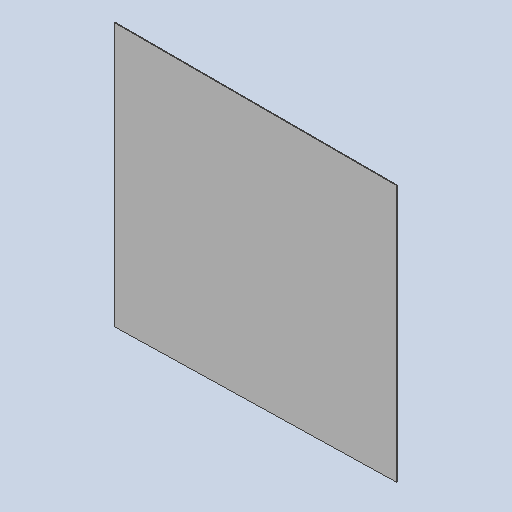
# Autodesk Inventor part: GBK 2311 shield 7
Saved by Autodesk Inventor 2026 (Build 300175000, 175)
## iProperties
Created: 2026-04-17
Part Number: GBK 2311 shield 7
Material: Steel
Document SubType Name: Sheet Metal
Designer: pokla
Stock Number: 2317
Mass: 69243.3 g
Surface Area: 44341.6 cm^2
Volume: 8820.8 cm^3
Density: 7.85 g/cm^3
Flat Pattern Width: 148 cm
Flat Pattern Length: 138.1 cm
Flat Pattern Area: 20438.8 cm^2
Sheet Metal Rule: По умолчанию_мм
Sheet Metal Width: 1480,000 мм
Sheet Metal Length: 1381,000 мм
Sheet Metal Area: 2043880,000 мм^2
Appearance: Default
Author: admin
Autodesk Inventor part; units mm, degrees
ref_plane "YZ Plane" through (0, 0, 0) normal (1, 0, 0) x (0, 1, 0)
ref_plane "XZ Plane" through (0, 0, 0) normal (0, 1, 0) x (-1, 0, 0)
ref_plane "XY Plane" through (0, 0, 0) normal (0, 0, 1) x (1, 0, 0)
sketch "Sketch1" plane through (0, 0, 0) normal (0, 0, 1) x (1, 0, 0)
  line L0 (740, -745) -> (-740, -745)
  line L1 (-740, -745) -> (-740, 745)
  line L2 (-740, 745) -> (740, 745)
  line L3 (740, 745) -> (740, -745)
  line L4 (740, -745) -> (-740, 745) construction
  line L5 (-740, -745) -> (740, 745) construction
  line L6 (-740, -636) -> (740, -602.4141)
  point P0 (0, 0)
  dimension "d0" = 1480
  dimension "d1" = 1490
  dimension "d4" = 1.3
  dimension "d9" = 1381
  dimension "d10" = 109
  measures "d0" distance of L1.end L2.end
  measures "d1" distance of L0.end L1.end
  measures "d4" angle of L0 L6
  measures "d9" distance of L1.end L6.start
  measures "d10" distance of L0.end L6.start
extrude "Plate1" add sketch "Sketch1" along normal blind 4 contours L6 L1 L2 L3
sketch "Эскиз3" plane through (0, 0, 0) normal (0, 0, -1) x (-1, 0, 0)
  line L0 (636.5062, -289.7957) -> (636.5062, -787.9319) construction
  line L1 (636.5062, -787.9319) -> (596.8789, -787.9319) construction
  line L2 (596.8789, -787.9319) -> (596.8789, -289.7957) construction
  line L3 (596.8789, -289.7957) -> (636.5062, -289.7957) construction
  line L4 (210.5058, -494) -> (210.5058, -591) projected
  line L5 (210.5058, -591) -> (206.5068, -591) projected
  line L6 (-289.6228, -494) -> (-289.6228, -591) projected
  line L7 (-289.6228, -591) -> (-293.6218, -591) projected
  line L8 (-739.3197, -490.5) -> (-710, -490.5) projected
  line L9 (-710, -490.5) -> (-710, -486.5) projected
  line L10 (-739.3197, 6.1667) -> (-710, 6.1667) projected
  line L11 (-710, 6.1667) -> (-710, 10.1667) projected
  line L12 (-739.3197, 502.8333) -> (-710, 502.8333) projected
  line L13 (-710, 502.8333) -> (-710, 506.8333) projected
  ellipse E0 centre (-289.6228, 744) end of major axis (-289.6228, 774) minor radius 0.6803 (-289.6228, 714) -> (-289.6228, 774) ccw projected
  line L14 (-289.6228, 714) -> (-293.6218, 714) projected
  ellipse E1 centre (210.5058, 744) end of major axis (210.5058, 774) minor radius 0.6803 (210.5058, 714) -> (210.5058, 774) ccw projected
  line L15 (210.5058, 714) -> (206.5068, 714) projected
  line L16 (710, -490.5) -> (710, -486.5) projected
  line L17 (710, 6.1667) -> (710, 10.1667) projected
  line L18 (710, 502.8333) -> (710, 506.8333) projected
  line L19 (710, -490.5) -> (680, -490.5)
  line L20 (710, 6.1667) -> (680, 6.1667)
  line L21 (710, 502.8333) -> (680, 502.8333)
  point P0 (0, 0)
  dimension "d11" = 30
  dimension "d12" = 30
  dimension "d13" = 30
  constraints: 6 end point, 3 horizontal, 4 other
  measures "d11" distance of L16.start L19.end
  measures "d12" distance of L20.start L20.end
  measures "d13" distance of L21.start L21.end
mark "Маркировка1"
equation "\"d0\" = Лист_ширина"
equation "\"d2\" = Thickness"
equation "\"BendRadius\" = Thickness"
equation "\"BendReliefWidth\" = Thickness"
equation "\"BendReliefDepth\" = 0.5 * Thickness"
equation "\"CornerReliefSize\" = 4 * Thickness"
equation "\"MinimumRemnant\" = 2 * Thickness"
equation "\"TransitionRadius\" = BendRadius"
equation "\"JacobiRadiusSize\" = BendRadius"
equation "\"GapSize\" = Thickness"
equation "\"Лист_ширина\" = 1480"
equation "\"Thickness\" = 4"
body "Solid1"
